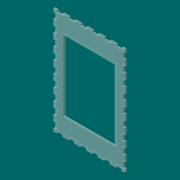
# Autodesk Inventor part: front
Saved by Autodesk Inventor 2016 (Build 200138000, 138)
## iProperties
Created: 2015-10-05
Part Number: front
Material: Polycarbonate, Clear
Document SubType Name: Modeling
Designer: Sawaiz
Density: 1.2 g/cm^3
Appearance: Polycarbonate - Clear
Author: Sawaiz
Autodesk Inventor part; units mm, degrees
ref_plane "YZ Plane" through (0, 0, 0) normal (1, 0, 0) x (0, 1, 0)
ref_plane "XZ Plane" through (0, 0, 0) normal (0, 1, 0) x (-1, 0, 0)
ref_plane "XY Plane" through (0, 0, 0) normal (0, 0, 1) x (1, 0, 0)
sketch "Sketch1" plane through (0, 0, 0) normal (0, 1, 0) x (-1, 0, 0)
  line L0 (60, -90) -> (-60, -90)
  line L1 (-60, -90) -> (-60, 90)
  line L2 (-60, 90) -> (60, 90)
  line L3 (60, 90) -> (60, -90)
  line L4 (60, -90) -> (-60, 90) construction
  line L5 (-60, -90) -> (60, 90) construction
  point P0 (0, 0)
  dimension "d0" = 120
  dimension "d1" = 180
  constraints: 12 end point, 2 midpoint, 2 parallel, 1 horizontal, 1 perpendicular
  measures "d0" distance of L1.end L2.end
  measures "d1" distance of L0.end L1.end
extrude "Extrusion1" add sketch "Sketch1" along normal blind 3.175
sketch "Sketch2" plane through (0, 0, 0) normal (0, -1, 0) x (1, 0, 0)
  line L0 (-43.8, -60) -> (43.8, -60)
  line L1 (43.8, -60) -> (43.8, 60)
  line L2 (43.8, 60) -> (-43.8, 60)
  line L3 (-43.8, 60) -> (-43.8, -60)
  line L4 (-43.8, -60) -> (43.8, 60) construction
  line L5 (43.8, -60) -> (-43.8, 60) construction
  line L6 (60, 90) -> (-60, 90) projected
  point P0 (0, 0)
  dimension "d4" = 87.6
  dimension "d8" = 30
  constraints: 12 end point, 2 midpoint, 2 parallel, 1 horizontal, 1 perpendicular
  measures "d4" distance of L2.end L1.end
  measures "d8" distance between parallel lines of L6 L2
extrude "Extrusion2" cut sketch "Sketch2" against normal through all
sketch "Sketch4" plane through (0, 0, 0) normal (0, -1, 0) x (1, 0, 0)
  line L0 (43.8, 60) -> (43.8, -60) projected
  line L1 (43.8, -60) -> (-43.8, -60) projected
  line L2 (-43.8, -60) -> (-43.8, 60) projected
  line L3 (-43.8, 60) -> (43.8, 60) projected
  line L4 (-60, -90) -> (60, -90) projected
  line L5 (60, -90) -> (60, 90) projected
  line L6 (60, 90) -> (-60, 90) projected
  line L7 (-60, 90) -> (-60, -90) projected
  line L8 (-60, 90) -> (60, 90) projected
  line L9 (-55, 90) -> (-45, 90)
  line L10 (-45, 90) -> (-45, 86.825)
  line L11 (-45, 86.825) -> (-55, 86.825)
  line L12 (-55, 86.825) -> (-55, 90)
  point P0 (0, 0)
  dimension "d25" = 10
  dimension "d26" = 5
  dimension "d27" = 3.175
  constraints: 8 end point, 2 parallel, 1 horizontal, 1 perpendicular, 1 point on line
  measures "d25" distance of L10.end L11.end
  measures "d26" distance between parallel lines of L7 L12
  measures "d27" distance of L11.end L9.start
extrude "Extrusion3" cut sketch "Sketch4" against normal through all contours L6 L10 L11 L12
pattern_linear "Rectangular Pattern1" count 6 spacing 20 along (1, 0, 0) of "Extrusion3"
mirror "Mirror1" about plane through (0, 0, 0) normal (0, 0, 1) of "Extrusion3", "Rectangular Pattern1"
sketch "Sketch5" plane through (0, 0, 0) normal (0, -1, 0) x (1, 0, 0)
  line L0 (55, -86.825) -> (55, -90) projected
  line L1 (55, -90) -> (60, -90) projected
  line L2 (60, -90) -> (60, 90) projected
  line L3 (60, 90) -> (55, 90) projected
  line L4 (55, 90) -> (55, 86.825) projected
  line L5 (55, 86.825) -> (45, 86.825) projected
  line L6 (45, 86.825) -> (45, 90) projected
  line L7 (45, 90) -> (35, 90) projected
  line L8 (35, 90) -> (35, 86.825) projected
  line L9 (35, 86.825) -> (25, 86.825) projected
  line L10 (25, 86.825) -> (25, 90) projected
  line L11 (25, 90) -> (15, 90) projected
  line L12 (15, 90) -> (15, 86.825) projected
  line L13 (15, 86.825) -> (5, 86.825) projected
  line L14 (5, 86.825) -> (5, 90) projected
  line L15 (5, 90) -> (-5, 90) projected
  line L16 (-5, 90) -> (-5, 86.825) projected
  line L17 (-5, 86.825) -> (-15, 86.825) projected
  line L18 (-15, 86.825) -> (-15, 90) projected
  line L19 (-15, 90) -> (-25, 90) projected
  line L20 (-25, 90) -> (-25, 86.825) projected
  line L21 (-25, 86.825) -> (-35, 86.825) projected
  line L22 (-35, 86.825) -> (-35, 90) projected
  line L23 (-35, 90) -> (-45, 90) projected
  line L24 (-45, 90) -> (-45, 86.825) projected
  line L25 (-45, 86.825) -> (-55, 86.825) projected
  line L26 (-55, 86.825) -> (-55, 90) projected
  line L27 (-55, 90) -> (-60, 90) projected
  line L28 (-60, 90) -> (-60, -90) projected
  line L29 (-60, -90) -> (-55, -90) projected
  line L30 (-55, -90) -> (-55, -86.825) projected
  line L31 (-55, -86.825) -> (-45, -86.825) projected
  line L32 (-45, -86.825) -> (-45, -90) projected
  line L33 (-45, -90) -> (-35, -90) projected
  line L34 (-35, -90) -> (-35, -86.825) projected
  line L35 (-35, -86.825) -> (-25, -86.825) projected
  line L36 (-25, -86.825) -> (-25, -90) projected
  line L37 (-25, -90) -> (-15, -90) projected
  line L38 (-15, -90) -> (-15, -86.825) projected
  line L39 (-15, -86.825) -> (-5, -86.825) projected
  line L40 (-5, -86.825) -> (-5, -90) projected
  line L41 (-5, -90) -> (5, -90) projected
  line L42 (5, -90) -> (5, -86.825) projected
  line L43 (5, -86.825) -> (15, -86.825) projected
  line L44 (15, -86.825) -> (15, -90) projected
  line L45 (15, -90) -> (25, -90) projected
  line L46 (25, -90) -> (25, -86.825) projected
  line L47 (25, -86.825) -> (35, -86.825) projected
  line L48 (35, -86.825) -> (35, -90) projected
  line L49 (35, -90) -> (45, -90) projected
  line L50 (45, -90) -> (45, -86.825) projected
  line L51 (45, -86.825) -> (55, -86.825) projected
  line L52 (43.8, 60) -> (43.8, -60) projected
  line L53 (43.8, -60) -> (-43.8, -60) projected
  line L54 (-43.8, -60) -> (-43.8, 60) projected
  line L55 (-43.8, 60) -> (43.8, 60) projected
  line L56 (60, 90) -> (60, -90) projected
  line L57 (60, 85) -> (56.825, 85)
  line L58 (56.825, 85) -> (56.825, 75)
  line L59 (56.825, 75) -> (60, 75)
  line L60 (60, 75) -> (60, 85)
  point P0 (0, 0)
  dimension "d33" = 3.175
  dimension "d34" = 5
  dimension "d35" = 10
  constraints: 8 end point, 2 parallel, 1 horizontal, 1 perpendicular, 1 point on line
  measures "d33" distance of L57.start L57.end
  measures "d34" distance between parallel lines of L3 L57
  measures "d35" distance between parallel lines of L57 L59
extrude "Extrusion4" cut sketch "Sketch5" against normal through all contours L59 L58 L57 L2
pattern_linear "Rectangular Pattern2" count 9 spacing 20 along (0, 0, -1) of "Extrusion4"
mirror "Mirror2" about plane through (0, 0, 0) normal (1, 0, 0) of "Extrusion4", "Rectangular Pattern2"
sketch "Sketch3" plane through (0, 0, 0) normal (0, -1, 0) x (1, 0, 0)
  line L0 (43.8, 60) -> (43.8, -60) projected
  line L1 (43.8, -65) -> (-43.8, -65) projected
  line L2 (-43.8, -60) -> (-43.8, 60) projected
  line L3 (-43.8, 65) -> (43.8, 65) projected
  line L4 (-60, -90) -> (60, -90) projected
  line L5 (60, -90) -> (60, 90) projected
  line L6 (60, 90) -> (-60, 90) projected
  line L7 (-60, 90) -> (-60, -90) projected
  line L8 (58.5014, 54) -> (58.5014, 18)
  line L9 (58.5014, 18) -> (-58.5014, 18)
  line L10 (-58.5014, 18) -> (-58.5014, 54)
  line L11 (-20, 88.5014) -> (-20, -88.5014)
  line L12 (-20, -88.5014) -> (20, -88.5014)
  line L13 (-43.8, 60) -> (-43.8, -60) projected
  line L14 (20, -88.5014) -> (20, 88.5014)
  line L15 (58.5014, -54) -> (58.5014, -18)
  line L16 (58.5014, -18) -> (-58.5014, -18)
  line L17 (-43.8, 60) -> (43.8, 60) projected
  line L18 (43.8, -60) -> (-43.8, -60) projected
  line L19 (-58.5014, -18) -> (-58.5014, 18)
  line L20 (-58.5014, -54) -> (-58.5014, -18)
  line L21 (58.5014, -18) -> (58.5014, 18)
  line L22 (-58.5014, -54) -> (58.5014, -54)
  line L23 (-58.5014, 54) -> (58.5014, 54)
  line L24 (-20, 88.5014) -> (20, 88.5014)
  point P0 (0, 0)
  dimension "d9" = 1.5875
  dimension "d10" = 1.5875
  dimension "d11" = 1.5875
  dimension "d12" = 1.5875
  dimension "d20" = 40
  dimension "d21" = 40
  dimension "d22" = 36
  dimension "d24" = 36
  constraints: 29 end point, 5 vertical, 3 collinear, 3 horizontal, 3 parallel, 2 perpendicular
  measures "d20" distance from line of L7 L11.start
  measures "d21" distance of L11.start L14.end
  measures "d22" distance from line of L4 L20.start
  measures "d24" distance of L20.start L16.end
equation "\"d0\" = width"
equation "\"d1\" = height"
equation "\"d2\" = materialThickness"
equation "\"d4\" = cardWidth + 4 * cardClearence"
equation "\"d6\" = materialThickness"
equation "\"d25\" = notchWidth"
equation "\"d26\" = 0.5 * notchWidth"
equation "\"d27\" = materialThickness"
equation "\"d32\" = 2 * notchWidth"
equation "\"d33\" = materialThickness"
equation "\"d34\" = 0.5 * notchWidth"
equation "\"d35\" = notchWidth"
equation "\"d40\" = 2 * notchWidth"
equation "\"d9\" = 0.5 * materialThickness"
equation "\"d10\" = 0.5 * materialThickness"
equation "\"d11\" = 0.5 * materialThickness"
equation "\"d12\" = 0.5 * materialThickness"
equation "\"d20\" = 0.333333 * width"
equation "\"d21\" = 0.333333 * width"
equation "\"d22\" = 0.2 * height"
equation "\"d24\" = 0.2 * height"
equation "\"height\" = 180"
equation "\"width\" = 120"
equation "\"materialThickness\" = 3.175"
equation "\"laserKerf\" = 0.1"
equation "\"cardPinDiameter\" = 3"
equation "\"spoolDiameter\" = 95"
equation "\"cardThickness\" = 0.76"
equation "\"cardFillet\" = 2.88"
equation "\"cardHeight\" = 53.98"
equation "\"cardSelected\" = 1"
equation "\"cardWidth\" = 85.6"
equation "\"centeralShaftDiameter\" = 8"
equation "\"cardClearence\" = 0.5"
equation "\"bearingOd\" = 22"
equation "\"bearingWidth\" = 8"
equation "\"axleHeight\" = 95"
equation "\"nutTrapClearence\" = 2"
equation "\"nutTrapwidth\" = 5.5"
equation "\"nutTrapDepth\" = 2.5"
equation "\"magnetDiameter\" = 6"
equation "\"magnetLength\" = 3"
equation "\"magnetProtusion\" = 0.25"
equation "\"notchWidth\" = 10"
equation "\"spoolThickness\" = 5.588"
body "Solid1"
